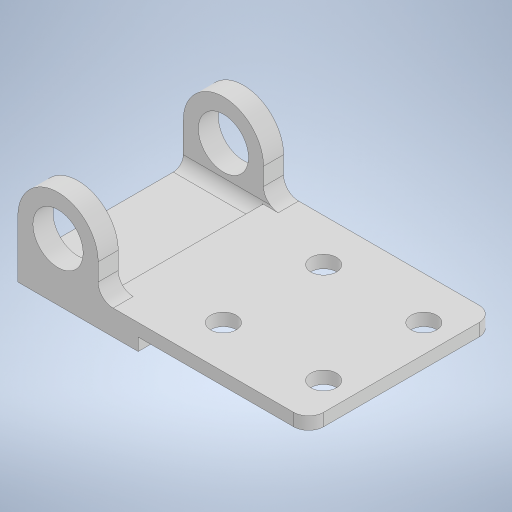
# Autodesk Inventor part: myBering
Saved by Autodesk Inventor 2023.1 (Build 271208000, 208)
## iProperties
Created: 2025-08-13
Part Number: myBering
Material: Типовые
Document SubType Name: Modeling
Designer: DELL
Density: 1 g/cm^3
Appearance: По умолчанию
Author: DELL
Autodesk Inventor part; units mm, degrees
ref_plane "YZ Plane" through (0, 0, 0) normal (1, 0, 0) x (0, 1, 0)
ref_plane "XZ Plane" through (0, 0, 0) normal (0, 1, 0) x (-1, 0, 0)
ref_plane "XY Plane" through (0, 0, 0) normal (0, 0, 1) x (1, 0, 0)
sketch "Эскиз1" plane through (0, 0, 0) normal (0, 0, 1) x (1, 0, 0)
  circle A0 centre (0, 8) radius 5
  line L0 (0, 0) -> (0, 16) construction
  circle A1 centre (0, 8) radius 8
  line L1 (8, 0) -> (8, 8)
  line L2 (-8, 8) -> (-8, 0)
  line L3 (-8, 0) -> (8, 0)
  dimension "d0" = 10
  dimension "d1" = 8
  dimension "d2" = 16
  constraints: 8 end point, 2 centre point, 2 coincident, 2 midpoint, 2 point on circle, 1 horizontal, 1 tangent, 1 vertical
  measures "d0" diameter of A0
  measures "d1" distance of L0.start A0.centre
  measures "d2" diameter of A1
extrude "Выдавливание1" add sketch "Эскиз1" along normal blind 4
sketch "Эскиз3" plane through (-8, 0, 0) normal (0, -1, 0) x (1, 0, 0)
  line L0 (0, 4) -> (16, 4)
  line L1 (16, 4) -> (16, -33)
  line L2 (16, -33) -> (0, -33)
  line L3 (0, -33) -> (0, 4)
  point P0 (8, 0)
  dimension "d5" = 16
  dimension "d6" = 37
  constraints: 8 end point, 2 parallel, 1 horizontal, 1 perpendicular
  measures "d5" distance of L1.end L2.end
  measures "d6" distance of L0.end L1.end
extrude "Выдавливание2" add sketch "Эскиз3" along normal blind 1
ref_plane "РабПлоскость1" through (8, 0, -14.5) normal (0, 0, -1) x (-1, 0, 0)
mirror "Зеркальное отражение2" about plane through (8, 0, -14.5) normal (0, 0, -1) of "Выдавливание1"
fillet "Сопряжение2" radius 2 1 edges at (0, 0, -29)
sketch "Эскиз6" plane through (-8, -1, 0) normal (0, -1, 0) x (1, 0, 0)
  line L0 (16, 4) -> (0, 4) projected
  line L1 (0, 4) -> (24, 4)
  line L2 (24, 4) -> (24, -33)
  line L3 (24, -33) -> (0, -33)
  line L4 (0, -33) -> (0, 4)
  point P0 (8, 0)
  dimension "d22" = 24
  dimension "d23" = 37
  constraints: 8 end point, 2 parallel, 1 horizontal, 1 perpendicular
  measures "d22" distance of L2.end L3.end
  measures "d23" distance of L1.end L2.end
extrude "Выдавливание5" add sketch "Эскиз6" along normal blind 2.5
sketch "Эскиз7" plane through (-8, -1, 0) normal (0, 1, 0) x (1, 0, 0)
  line L0 (16, 33) -> (24, 33) projected
  line L1 (16, 33) -> (58, 33)
  line L2 (58, 33) -> (58, -4)
  line L3 (58, -4) -> (16, -4)
  line L4 (16, -4) -> (16, 33)
  point P0 (8, 0)
  dimension "d26" = 42
  constraints: 8 end point, 2 parallel, 1 horizontal, 1 perpendicular
  measures "d26" distance of L2.end L3.end
extrude "Выдавливание6" add sketch "Эскиз7" along normal blind 2.5
sketch "Эскиз8" plane through (-8, 0, 0) normal (0, 1, 0) x (1, 0, 0)
  circle A0 centre (52.5, 24.5) radius 2.55
  circle A1 centre (32.5, 24.5) radius 2.55
  circle A2 centre (52.5, 4.5) radius 2.55
  circle A3 centre (32.5, 4.5) radius 2.55
  line L0 (16, -4) -> (58, -4) projected
  line L1 (58, -4) -> (58, 33) projected
  line L2 (58, 33) -> (16, 33) projected
  point P0 (8, 0)
  dimension "d29" = 8.5
  dimension "d30" = 5.5
  dimension "d31" = 5.1
  dimension "d32" = 5.5
  dimension "d33" = 8.5
  constraints: 4 centre point
  measures "d29" distance from line of L0 A2.centre
  measures "d30" distance from line of L1 A2.centre
  measures "d31" diameter of A2
  measures "d32" distance from line of L1 A0.centre
  measures "d33" distance from line of L2 A0.centre
extrude "Выдавливание7" cut sketch "Эскиз8" against normal blind 2.5
fillet "Сопряжение4" radius 3 2 edges at (50, 0.25, 4) (50, 0.25, -33)
fillet "Сопряжение6" radius 3 2 edges at (8, 1.5, -30.9682) (8, 1.5, 2)
sketch "Эскиз10" plane through (-8, 1.5, 0) normal (0, 1, 0) x (1, 0, 0)
  circle A0 centre (52.5, 4.5) radius 2.55 projected
  circle A1 centre (52.5, 24.5) radius 2.55 projected
  circle A2 centre (32.5, 24.5) radius 2.55 projected
  circle A3 centre (32.5, 4.5) radius 2.55 projected
  point P0 (8, 0)
extrude "Выдавливание8" cut sketch "Эскиз10" against normal blind 10
fillet "Сопряжение грани1" radius 0.15 1 edges at (8, 0, -13.5)
